Hager Rail Safe (Autodesk Fusion 360 design; units mm, degrees)
Autodesk Fusion 360 part; units mm, degrees
sketch "Sketch1" plane through (0, 0, 0) normal (0, 0, 1) x (1, 0, 0)
  line L0 (0, 0) -> (87, 0)
  line L1 (87, 0) -> (87, 1.4)
  line L2 (87, 1.4) -> (0, 1.4)
  line L3 (0, 1.4) -> (0, 0)
  line L4 (0, 1.4) -> (87, 1.4)
  line L5 (87, 1.4) -> (87, 2.8)
  line L6 (87, 2.8) -> (0, 2.8)
  line L7 (0, 2.8) -> (0, 1.4)
  line L8 (0, 0) -> (87, 0)
  line L9 (87, 0) -> (87, -1.4)
  line L10 (87, -1.4) -> (0, -1.4)
  line L11 (0, -1.4) -> (0, 0)
  dimension "d1" = 1.4
  dimension "d2" = 87
  dimension "d3" = 1.4
  dimension "d4" = 1.4
  constraint horizontal L0
  constraint vertical L1
  constraint horizontal L2
  constraint vertical L3
  constraint coincident L0.start L3.end
  constraint horizontal L4
  constraint vertical L5
  constraint horizontal L6
  constraint vertical L7
  constraint horizontal L8
  constraint vertical L9
  constraint horizontal L10
  constraint vertical L11
  measures "d1" distance of L0.start L2.end
  measures "d2" distance of L1.end L2.end
  measures "d3" distance of L2.end L6.end
  measures "d4" distance of L0.start L10.end
extrude "Extrude1" add sketch "Sketch1" along normal blind 1.4
extrude "Extrude2" add sketch "Sketch1" along normal blind 11 contours L0 L8 L9 L10 L11 | L2 L4 L5 L6 L7
